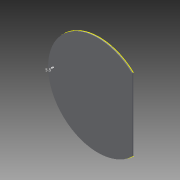
# Autodesk Inventor part: PCB
Saved by Autodesk Inventor 2015 (Build 190159000, 159)
## iProperties
Created: 2016-09-07
Part Number: PCB
Material: Generic
Document SubType Name: Modeling
Designer: James Yelland
Density: 1 g/cm^3
Appearance: Default
Author: James Yelland
Autodesk Inventor part; units mm, degrees
ref_plane "YZ Plane" through (0, 0, 0) normal (1, 0, 0) x (0, 1, 0)
ref_plane "XZ Plane" through (0, 0, 0) normal (0, 1, 0) x (-1, 0, 0)
ref_plane "XY Plane" through (0, 0, 0) normal (0, 0, 1) x (1, 0, 0)
sketch "Sketch1" plane through (0, 0, 0) normal (0, 1, 0) x (-1, 0, 0)
  line L0 (0, 0) -> (-55, 0)
  line L1 (-55, 0) -> (-55, -58.0948)
  line L2 (-55, 0) -> (-55, 58.0948)
  arc A0 (-55, -58.0948) -> (-55, 58.0948) centre (0, 0) ccw
  dimension "d1" = 55
  constraints: 6 end point, 2 coincident, 2 point on circle, 1 centre point, 1 horizontal, 1 perpendicular, 1 point on line
  measures "d1" distance of L0.start L0.end
extrude "Extrusion1" add sketch "Sketch1" along normal blind 2
sketch "Sketch2" plane through (0, 2, 0) normal (0, 1, 0) x (1, 0, 0)
  point P0 (0, 0)
sketch "Sketch3" plane through (0, 2, 0) normal (0, 1, 0) x (1, 0, 0)
  line L0 (-75.95, 0) -> (-75.95, 5)
  line L1 (-75.95, 5) -> (-71.95, 5)
  line L2 (-71.95, 5) -> (-71.95, -5)
  line L3 (-71.95, -5) -> (-75.95, -5)
  line L4 (-75.95, -5) -> (-75.95, 0)
  line L5 (-75.95, 0) -> (-77.75, 0)
  line L6 (-77.75, 0) -> (-75, 0)
  line L7 (-75, 0) -> (-80, 0)
  arc A0 (55, 58.0948) -> (55, -58.0948) centre (0, 0) ccw projected
  circle A1 centre (-75, 0) radius 2.75
  dimension "d12" = 5.5
  constraints: 16 end point, 4 perpendicular, 2 coincident, 1 centre point, 1 horizontal, 1 point on line, 1 vertical
  measures "d12" diameter of A1
body "Solid1"
